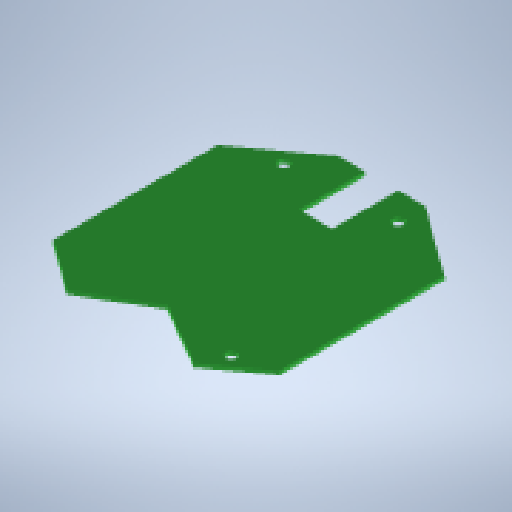
# Autodesk Inventor part: PCB
Saved by Autodesk Inventor 2024 (Build 280153000, 153)
## iProperties
Created: 2023-11-11
Part Number: PCB
Material: FR4
Document SubType Name: Modeling
Designer: jevan
Density: 1 g/cm^3
Appearance: Generic
Author: jevan
Autodesk Inventor part; units mm, degrees
ref_plane "YZ Plane" through (0, 0, 0) normal (1, 0, 0) x (0, 1, 0)
ref_plane "XZ Plane" through (0, 0, 0) normal (0, 1, 0) x (-1, 0, 0)
ref_plane "XY Plane" through (0, 0, 0) normal (0, 0, 1) x (1, 0, 0)
sketch "Sketch1" plane through (0, 0, 0) normal (0, 0, 1) x (1, 0, 0)
  line L0 (9.734, 29.9583) -> (25.484, 18.5152)
  line L1 (25.484, 18.5152) -> (31.5, 0)
  line L2 (31.5, 0) -> (25.484, -18.5152)
  line L3 (25.484, -18.5152) -> (9.734, -29.9583)
  line L4 (9.734, -29.9583) -> (-9.734, -29.9583)
  line L5 (-9.734, -29.9583) -> (-25.484, -18.5152)
  line L6 (-25.484, -18.5152) -> (-31.5, 0)
  line L7 (-31.5, 0) -> (-25.484, 18.5152)
  line L8 (-25.484, 18.5152) -> (-9.734, 29.9583)
  line L9 (-9.734, 29.9583) -> (9.734, 29.9583)
  line L10 (0, 29.9583) -> (0, 0)
  line L11 (-13.8564, 26.9632) -> (0, 18.9632)
  line L12 (0, 18.9632) -> (13.8564, 26.9632)
  line L13 (-23.3574, 16.9702) -> (-28.8713, 0)
  line L14 (-28.8713, 0) -> (-23.3574, -16.9702)
  line L15 (-23.3574, -16.9702) -> (-8.9217, -27.4583)
  line L16 (-8.9217, -27.4583) -> (8.9217, -27.4583)
  line L17 (8.9217, -27.4583) -> (23.3574, -16.9702)
  line L18 (23.3574, -16.9702) -> (28.8713, 0)
  line L19 (28.8713, 0) -> (23.3574, 16.9702)
  line L20 (8.9217, 27.4583) -> (-8.9217, 27.4583)
  line L21 (-8.9217, 27.4583) -> (-11.4864, 25.5949)
  line L22 (-12.9919, 24.5011) -> (-23.3574, 16.9702)
  line L23 (-12.9919, 24.5011) -> (0, 17.0002)
  line L24 (23.3574, 16.9702) -> (12.9919, 24.5011)
  line L25 (11.4864, 25.5949) -> (8.9217, 27.4583)
  line L26 (0, 17.0002) -> (12.9919, 24.5011)
  line L27 (0, 16.7115) -> (-12.9763, 24.2034)
  line L28 (-12.9763, 24.2034) -> (-23.1447, 16.8156)
  line L29 (-23.1447, -16.8156) -> (-8.8405, -27.2083)
  line L30 (8.8405, -27.2083) -> (23.1447, -16.8156)
  line L31 (23.1447, 16.8156) -> (12.9763, 24.2034)
  line L32 (12.9763, 24.2034) -> (0, 16.7115)
  line L33 (-23.1447, 16.8156) -> (-23.1447, -16.8156)
  line L34 (23.1447, 16.8156) -> (23.1447, -16.8156)
  line L35 (-3.35, -27.2083) -> (-3.35, -13.7083)
  line L36 (-3.35, -13.7083) -> (3.35, -13.7083)
  line L37 (3.35, -13.7083) -> (3.35, -27.2083)
  line L38 (-8.8405, -27.2083) -> (-3.35, -27.2083)
  line L39 (3.35, -27.2083) -> (8.8405, -27.2083)
  circle A0 centre (15.4447, 19.0034) radius 3
  circle A1 centre (15.4447, 19.0034) radius 1.1
  circle A2 centre (-13.15, -20.3083) radius 3
  circle A3 centre (-13.15, -20.3083) radius 1.1
  circle A4 centre (8.85, -21.7083) radius 3
  circle A5 centre (8.85, -21.7083) radius 1.1
  circle A6 centre (15.4447, 19.0034) radius 2
  circle A7 centre (-13.15, -20.3083) radius 2
  circle A8 centre (8.85, -21.7083) radius 2
  dimension "d0" = 63
  dimension "d1" = 16
  dimension "d4" = 120
  dimension "d6" = 2.5
  dimension "d7" = 1.7
  dimension "d8" = 0.25
  dimension "d11" = 6.7
  dimension "d12" = 13.5
  dimension "d13" = 0.25
  dimension "d15" = 0.25
  dimension "d16" = 0.25
  dimension "d24" = 6
  dimension "d25" = 2.2
  dimension "d26" = 6
  dimension "d27" = 2.2
  dimension "d28" = 6
  dimension "d29" = 2.2
  dimension "d30" = 5.5
  dimension "d31" = 5.5
  dimension "d32" = 9.8
  dimension "d33" = 6.9
  dimension "d36" = 5.2
  dimension "d37" = 7.7
  dimension "d38" = 4
  dimension "d39" = 4
  dimension "d40" = 4
  constraints: 80 end point, 11 equal length, 9 centre point, 7 coincident, 6 parallel, 5 point on line, 3 collinear, 2 vertical, 1 horizontal, 1 midpoint, 1 perpendicular, 29 other
  measures "d0" distance of L1.end L6.end
  measures "d1" distance of L11.start L11.end
  measures "d4" angle of L12 L11
  measures "d6" distance between parallel lines of L8 L22
  measures "d7" distance between parallel lines of L11 L23
  measures "d8" distance between parallel lines of L23 L27
  measures "d11" distance of L35.end L36.end
  measures "d12" distance of L35.start L35.end
  measures "d13" distance between parallel lines of L30 L17
  measures "d15" distance from line of L14 L29.start
  measures "d16" distance between parallel lines of L38 L16
  measures "d24" diameter of A0
  measures "d25" diameter of A1
  measures "d26" diameter of A2
  measures "d27" diameter of A3
  measures "d28" diameter of A4
  measures "d29" diameter of A5
  measures "d30" distance from line of L39 A4.centre
  measures "d31" distance from line of L37 A4.centre
  measures "d32" distance from line of A2.centre L35
  measures "d33" distance from line of L38 A3.centre
  measures "d36" vertical distance of L31.end A1.centre
  measures "d37" distance from line of L34 A1.centre
  measures "d38" diameter of A6
  measures "d39" diameter of A7
  measures "d40" diameter of A8
extrude "Extrusion1" add sketch "Sketch1" along normal blind 0.8 contours L32 L31 A0 L34 L30 L39 L37 L36 L35 L38 L29 L33 L28 L27 | L31 A0 | A2 | A4 | A6 | A7 | A8 picked at (16.9034, 21.0385)
body "Solid1"
